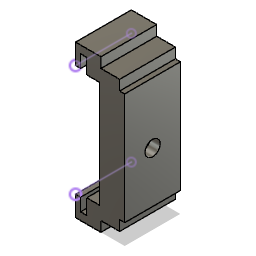
encoche v3 (Autodesk Fusion 360 design; units mm, degrees)
Autodesk Fusion 360 part; units mm, degrees
sketch "Esquisse1" plane through (0, 0, 0) normal (0, 0, 1) x (1, 0, 0)
  line L0 (0, 4) -> (0, 0)
  line L1 (0, 0) -> (5, 0)
  line L2 (5, 0) -> (5, 2)
  line L3 (5, 2) -> (8.7, 2)
  line L4 (8.7, 2) -> (8.7, 4)
  line L5 (8.7, 4) -> (9.7, 4)
  line L6 (9.7, 4) -> (9.7, 26)
  line L7 (9.7, 26) -> (8.7, 26)
  line L8 (8.7, 26) -> (8.7, 28)
  line L9 (8.7, 28) -> (5, 28)
  line L10 (5, 28) -> (5, 30)
  line L11 (5, 30) -> (0, 30)
  line L12 (0, 30) -> (0, 26)
  line L13 (0, 26) -> (1, 26)
  line L14 (1, 26) -> (1, 28.5)
  line L15 (1, 28.5) -> (2.2, 28.5)
  line L16 (2.2, 28.5) -> (2.2, 25.5)
  line L17 (2.2, 25.5) -> (4.7, 25.5)
  line L18 (4.7, 25.5) -> (4.7, 4.5)
  line L19 (4.7, 4.5) -> (2.2, 4.5)
  line L20 (2.2, 4.5) -> (2.2, 1.5)
  line L21 (2.2, 1.5) -> (1, 1.5)
  line L22 (1, 1.5) -> (1, 4)
  line L23 (1, 4) -> (0, 4)
  dimension "d1" = 4
  dimension "d2" = 1.2
  dimension "d3" = 1
  dimension "d4" = 21
  dimension "d5" = 1.5
  dimension "d6" = 5
  dimension "d7" = 30
  dimension "d8" = 2.5
  dimension "d9" = 2
  dimension "d10" = 2
  dimension "d11" = 5
  dimension "d12" = 1
  constraint coincident L0.end L1.start
  constraint vertical L0
  constraint perpendicular L0 L1
  constraint perpendicular L1 L2
  constraint perpendicular L2 L3
  constraint perpendicular L3 L4
  constraint perpendicular L4 L5
  constraint perpendicular L3 L6
  constraint perpendicular L6 L7
  constraint perpendicular L7 L8
  constraint perpendicular L8 L9
  constraint perpendicular L9 L10
  constraint perpendicular L10 L11
  constraint perpendicular L11 L12
  constraint perpendicular L12 L13
  constraint perpendicular L13 L14
  constraint perpendicular L14 L15
  constraint perpendicular L15 L16
  constraint perpendicular L16 L17
  constraint perpendicular L17 L18
  constraint perpendicular L18 L19
  constraint perpendicular L19 L20
  constraint perpendicular L20 L21
  constraint perpendicular L21 L22
  constraint perpendicular L0 L23
  constraint equal L0 L12
  constraint equal L14 L22
  constraint equal L13 L23
  constraint equal L1 L11
  constraint equal L2 L10
  constraint equal L17 L19
  constraint equal L15 L21
  constraint equal L16 L20
  constraint equal L3 L9
  constraint equal L4 L8
  measures "d1" distance of L11.end L12.end
  measures "d2" distance of L20.end L21.end
  measures "d3" distance of L12.end L13.end
  measures "d4" distance of L17.end L18.end
  measures "d5" distance of L11 L15
  measures "d6" distance of L10.end L11.end
  measures "d7" distance of L1 L11
  measures "d8" distance of L16.end L17.end
  measures "d9" distance of L9.end L10.end
  measures "d10" distance of L3.end L4.end
  measures "d11" distance of L6 L18
  measures "d12" distance of L4.end L5.end
extrude "Extrusion1" add sketch "Esquisse1" along normal blind 11
sketch "Esquisse2" plane through (0, 0, 0) normal (1, 0, 0) x (0, 0, -1)
  line L0 (0, 26) -> (-11, 26)
  line L1 (0, 4) -> (-11, 4)
sketch "Esquisse3" plane through (0, 0, 0) normal (1, 0, 0) x (0, 0, -1)
sketch "Esquisse4" plane through (4.7, 0, 0) normal (-1, 0, 0) x (0, 0, 1)
  line L0 (0, 25.5) -> (0, 4.5)
  line L1 (0, 4.5) -> (11, 4.5)
  line L2 (11, 4.5) -> (11, 25.5)
  line L3 (11, 25.5) -> (0, 25.5)
  line L4 (0, 26) -> (11, 26)
  line L5 (0, 4) -> (11, 4)
  circle A0 centre (5.5, 14) radius 1.5
  dimension "d16" = 3
  measures "d16" diameter of A0
sketch "Esquisse5" plane through (4.7, 0, 0) normal (-1, 0, 0) x (0, 0, 1)
  line L0 (0, 25.5) -> (0, 4.5)
  line L1 (0, 4.5) -> (11, 4.5)
  line L2 (11, 4.5) -> (11, 25.5)
  line L3 (11, 25.5) -> (0, 25.5)
  circle A0 centre (5.5, 14) radius 1.5
  dimension "d27" = 3
  measures "d27" diameter of A0
hole "Perçage3" at (4.7, 14, 5.5) direction (1, 0, 0) diameter 3 depth 5 tip angle 180 counterbore diameter 5 counterbore depth 3
sketch "Esquisse6" plane through (0, 0, 0) normal (0, 0, 1) x (1, 0, 0)
hole "Perçage1" [suppressed]
hole "Perçage2" [suppressed]
